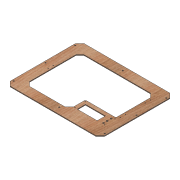
# Autodesk Inventor part: Front Face
Saved by Autodesk Inventor 2015 (Build 190159000, 159)
## iProperties
Created: 2018-04-12
Part Number: Front Face
Material: Wood (Birch)
Document SubType Name: Modeling
Designer: Ghassan Yusuf
Density: 0.55 g/cm^3
Appearance: Birch - Natural Polished
Author: Ghassan Yusuf
Autodesk Inventor part; units mm, degrees
ref_plane "YZ Plane" through (0, 0, 0) normal (1, 0, 0) x (0, 1, 0)
ref_plane "XZ Plane" through (0, 0, 0) normal (0, 1, 0) x (-1, 0, 0)
ref_plane "XY Plane" through (0, 0, 0) normal (0, 0, 1) x (1, 0, 0)
sketch "Faces Holing" plane through (0, 0, 0) normal (0, 0, 1) x (1, 0, 0)
  circle A0 centre (-222, 150) radius 3
  circle A1 centre (-222, 5) radius 3
  circle A2 centre (-222, -150) radius 3
  circle A3 centre (222, -150) radius 3
  circle A4 centre (222, 5) radius 3
  circle A5 centre (222, 150) radius 3
  circle A6 centre (0, 160) radius 3
  circle A7 centre (0, -150) radius 3
  point P0 (0, 2.5)
  dimension "d22" = 6
  dimension "d23" = 145
  dimension "d24" = 155
  measures "d22" diameter of A0
  measures "d23" distance of A4.centre A5.centre
  measures "d24" distance of A3.centre A4.centre
sketch "Hinges" plane through (0, 0, 0) normal (0, 0, 1) x (1, 0, 0)
  circle A0 centre (-439.8647, 121.4101) radius 1.75
  circle A1 centre (-439.8647, 95.9101) radius 1.75
  line L0 (-433.3647, 128.6601) -> (-449.3647, 128.6601)
  line L1 (-449.3647, 128.6601) -> (-449.3647, 88.6601)
  line L2 (-449.3647, 88.6601) -> (-433.3647, 88.6601)
  line L3 (-433.3647, 88.6601) -> (-433.3647, 128.6601)
  circle A2 centre (-464.8647, 95.9101) radius 1.75
  circle A3 centre (-464.8647, 121.4101) radius 1.75
  line L4 (-471.3647, 88.6601) -> (-455.3647, 88.6601)
  line L5 (-455.3647, 88.6601) -> (-455.3647, 128.6601)
  line L6 (-455.3647, 128.6601) -> (-471.3647, 128.6601)
  line L7 (-471.3647, 128.6601) -> (-471.3647, 88.6601)
  point P0 (-452.3647, 108.6601)
  dimension "d35" = 3.5
  dimension "d36" = 25.5
  dimension "d37" = 6.5
  dimension "d38" = 40
  dimension "d39" = 7.25
  dimension "d40" = 16
  dimension "d41" = 3.5
  dimension "d42" = 25.5
  dimension "d43" = 6.5
  dimension "d44" = 40
  dimension "d45" = 7.25
  dimension "d46" = 16
  dimension "d47" = 38
  measures "d35" diameter of A0
  measures "d36" distance of A1.centre A0.centre
  measures "d37" distance from line of L3 A0.centre
  measures "d38" distance of L2.end L0.start
  measures "d39" distance from line of L2 A1.centre
  measures "d40" distance of L0.start L0.end
  measures "d41" diameter of A2
  measures "d42" distance of A3.centre A2.centre
  measures "d43" distance from line of L7 A2.centre
  measures "d44" distance of L6.end L4.start
  measures "d45" distance from line of L6 A3.centre
  measures "d46" distance of L4.start L4.end
  measures "d47" distance between parallel lines of L3 L7
sketch "LCD2004" plane through (0, 0, 0) normal (0, 0, 1) x (1, 0, 0)
  line L0 (36.575, 21.45) -> (-61.225, 21.45)
  line L1 (-61.225, 21.45) -> (-61.225, -19.15)
  line L2 (-61.225, -19.15) -> (36.575, -19.15)
  line L3 (36.575, -19.15) -> (36.575, 21.45)
  circle A0 centre (-72.4, 31.74) radius 1.7
  circle A1 centre (-72.4, -18.56) radius 1.7
  circle A2 centre (72.4, -18.56) radius 1.7
  circle A3 centre (72.4, 31.74) radius 1.7
  line L4 (59.475, -39.15) -> (79.475, -19.15)
  circle A4 centre (61.875, 23.63) radius 4
  circle A5 centre (61.875, 4.43) radius 4
  circle A6 centre (61.875, -13.37) radius 4
  line L5 (-79.475, -39.15) -> (59.475, -39.15)
  line L6 (79.475, -19.15) -> (79.475, 39.15)
  line L7 (79.475, 39.15) -> (-79.475, 39.15)
  line L8 (-79.475, 39.15) -> (-79.475, -39.15)
  line L9 (-79.475, -39.15) -> (79.475, 39.15) construction
  line L10 (79.475, -39.15) -> (-79.475, 39.15) construction
  line L11 (-60.925, 21.15) -> (36.275, 21.15)
  line L12 (36.275, 21.15) -> (36.275, -18.85)
  line L13 (36.275, -18.85) -> (-60.925, -18.85)
  line L14 (-60.925, -18.85) -> (-60.925, 21.15)
  line L15 (-60.925, 21.15) -> (36.275, -18.85) construction
  line L16 (36.275, 21.15) -> (-60.925, -18.85) construction
  point P0 (4.405, 0.2073)
  point P1 (-12.325, 1.15)
  dimension "d55" = 158.95
  dimension "d56" = 78.3
  dimension "d57" = 18.55
  dimension "d58" = 20.3
  dimension "d59" = 20
  dimension "d60" = 8
  dimension "d61" = 8
  dimension "d62" = 8
  dimension "d63" = 40
  dimension "d64" = 97.2
  dimension "d65" = 15.52
  dimension "d66" = 17.6
  dimension "d67" = 19.2
  dimension "d68" = 17.8
  dimension "d69" = 3.4
  dimension "d70" = 50.3
  dimension "d71" = 7.41
  dimension "d72" = 7.075
  dimension "d73" = 144.8
  dimension "d74" = 0.3
  dimension "d75" = 20
  measures "d55" distance of L6.end L7.end
  measures "d56" distance between parallel lines of L5 L7
  measures "d57" distance between parallel lines of L8 L14
  measures "d58" distance between parallel lines of L5 L13
  measures "d59" distance from line of L4.start L6
  measures "d60" diameter of A4
  measures "d61" diameter of A5
  measures "d62" diameter of A6
  measures "d63" distance between parallel lines of L13 L11
  measures "d64" distance between parallel lines of L12 L14
  measures "d65" distance from line of L7 A4.centre
  measures "d66" distance from line of L6 A4.centre
  measures "d67" distance of A5.centre A4.centre
  measures "d68" distance of A6.centre A5.centre
  measures "d69" diameter of A0
  measures "d70" distance of A1.centre A0.centre
  measures "d71" distance from line of L7 A0.centre
  measures "d72" distance from line of L8 A0.centre
  measures "d73" distance of A3.centre A0.centre
  measures "d74" distance between parallel lines of L11 L0
  measures "d75" distance from line of L5 L4.end
sketch "Door Shape" plane through (0, 0, 0) normal (0, 0, 1) x (1, 0, 0)
  line L0 (13.05, -134) -> (33.05, -114)
  line L1 (33.05, -114) -> (33.05, -55.7)
  line L2 (33.05, -55.7) -> (182, -55.7)
  line L3 (182, -55.7) -> (182, 113)
  line L4 (182, 113) -> (162, 133)
  line L5 (162, 133) -> (-162, 133)
  line L6 (-162, 133) -> (-182, 113)
  line L7 (-182, 113) -> (-182, -114)
  line L8 (-182, -114) -> (-162, -134)
  line L9 (-162, -134) -> (13.05, -134)
  point P0 (-8.285, -11.54)
sketch "Sketch1" plane through (0, 0, 0) normal (0, 0, 1) x (1, 0, 0)
  line L0 (-230, 180) -> (230, 180)
  line L1 (230, 180) -> (230, -180)
  line L2 (230, -180) -> (-230, -180)
  line L3 (-230, -180) -> (-230, 180)
  line L4 (-182, 133) -> (182, 133)
  line L5 (182, 133) -> (182, -49)
  line L6 (-18, -134) -> (-182, -134)
  line L7 (-182, -134) -> (-182, 133)
  line L8 (-18, -134) -> (33.05, -134)
  line L9 (182, -55.7) -> (182, -49)
  line L10 (33.05, -55.7) -> (182, -55.7)
  line L11 (33.05, -134) -> (33.05, -55.7)
  point P0 (0, 0)
  point P1 (0, 180)
  point P2 (-230, 0)
  point P3 (0, 133)
  dimension "d0" = 360
  dimension "d1" = 460
  dimension "d5" = 364
  dimension "d6" = 267
  dimension "d53" = 148.95
  dimension "d54" = 78.3
  constraints: 24 end point, 4 horizontal, 4 perpendicular, 3 midpoint, 3 parallel, 2 vertical alignment, 1 horizontal alignment
  measures "d0" distance of L2.end L0.start
  measures "d1" distance of L0.start L0.end
  measures "d5" distance between parallel lines of L5 L7
  measures "d6" distance between parallel lines of L6 L4
  measures "d53" distance between parallel lines of L9 L11
  measures "d54" distance between parallel lines of L8 L10
extrude "Extrusion1" add sketch "Sketch1" against normal blind 4
chamfer "Chamfer1" distance 20 angle 45 4 edges at (230, 180, -2) (-230, 180, -2) (-230, -180, -2) (230, -180, -2)
chamfer "Chamfer2" distance 20 angle 45 4 edges at (-182, -134, -2) (-182, 133, -2) (182, 133, -2) (33.05, -134, -2)
sketch "Sketch3" plane through (0, 0, 0) normal (0, 0, 1) x (1, 0, 0)
  line L0 (210, -180) -> (-210, -180) projected
  line L1 (-230, -160) -> (-230, 160) projected
  line L2 (230, -160) -> (230, 160) projected
  line L3 (-210, 180) -> (210, 180) projected
  circle A0 centre (-222, 150) radius 3
  circle A1 centre (-222, 5) radius 3
  circle A2 centre (-222, -150) radius 3
  circle A3 centre (222, -150) radius 3
  circle A4 centre (222, 5) radius 3
  circle A5 centre (222, 150) radius 3
  circle A6 centre (0, 160) radius 3
  circle A7 centre (0, -150) radius 3
  point P0 (0, 0)
  dimension "d25" = 30
  dimension "d29" = 30
  dimension "d30" = 20
  dimension "d31" = 230
  dimension "d32" = 230
  measures "d31" distance of the line from the sketch origin of L1
  measures "d32" distance of the line from the sketch origin of L1
extrude "Extrusion3" cut sketch "Sketch3" against normal blind 46.25
sketch "Sketch4" plane through (0, 0, 0) normal (0, 0, 1) x (1, 0, 0)
  line L0 (-182, -114) -> (-182, 113) projected
  line L1 (182, -55.7) -> (182, 113) projected
  line L2 (33.05, -55.7) -> (182, -55.7) projected
  line L3 (162, 133) -> (-162, 133) projected
  circle A0 centre (191.5, 103.6789) radius 1.75
  circle A1 centre (191.5, 78.1789) radius 1.75
  line L4 (198, 110.9289) -> (182, 110.9289)
  line L5 (182, 110.9289) -> (182, 70.9289)
  line L6 (182, 70.9289) -> (198, 70.9289)
  line L7 (198, 70.9289) -> (198, 110.9289)
  circle A2 centre (166.5, 78.1789) radius 1.75
  circle A3 centre (166.5, 103.6789) radius 1.75
  line L8 (160, 70.9289) -> (176, 70.9289)
  line L9 (176, 70.9289) -> (176, 110.9289)
  line L10 (176, 110.9289) -> (160, 110.9289)
  line L11 (160, 110.9289) -> (160, 70.9289)
  circle A4 centre (191.5, -17.95) radius 1.75
  circle A5 centre (191.5, -43.45) radius 1.75
  line L12 (198, -10.7) -> (182, -10.7)
  line L13 (182, -10.7) -> (182, -50.7)
  line L14 (182, -50.7) -> (198, -50.7)
  line L15 (198, -50.7) -> (198, -10.7)
  circle A6 centre (166.5, -43.45) radius 1.75
  circle A7 centre (166.5, -17.95) radius 1.75
  line L16 (160, -50.7) -> (176, -50.7)
  line L17 (176, -50.7) -> (176, -10.7)
  line L18 (176, -10.7) -> (160, -10.7)
  line L19 (160, -10.7) -> (160, -50.7)
  circle A8 centre (-166.5, 12.75) radius 1.75
  circle A9 centre (-166.5, -12.75) radius 1.75
  line L20 (-160, 20) -> (-176, 20)
  line L21 (-176, 20) -> (-176, -20)
  line L22 (-176, -20) -> (-160, -20)
  line L23 (-160, -20) -> (-160, 20)
  circle A10 centre (-191.5, -12.75) radius 1.75
  circle A11 centre (-191.5, 12.75) radius 1.75
  line L24 (-198, -20) -> (-182, -20)
  line L25 (-182, -20) -> (-182, 20)
  line L26 (-182, 20) -> (-198, 20)
  line L27 (-198, 20) -> (-198, -20)
  point P0 (0, 0)
  point P1 (-182, -111.9289)
  point P2 (-182, 110.9289)
  point P3 (-160, 0)
  point P4 (182, 110.9289)
  point P5 (38.05, -55.7)
  point P6 (159.9289, 133)
  point P7 (-159.9289, 133)
  point P8 (182, -50.7)
  point P9 (177, -55.7)
  dimension "d77" = 5
  dimension "d81" = 10.7
  dimension "d82" = 70.9289
  dimension "d83" = 78.1789
  dimension "d84" = 17.95
  constraints: 3 vertical, 1 horizontal alignment, 2 other
extrude "Extrusion4" cut sketch "Sketch4" against normal blind 10 contours A0 | A1 | A4 | A5 | A10 | A11
fillet "Fillet2" radius 5 8 edges at (-210, -180, -2) (-230, -160, -2) (-230, 160, -2) (-210, 180, -2) (210, 180, -2) (230, 160, -2) (210, -180, -2) (230, -160, -2)
sketch "Sketch5" plane through (0, 0, 0) normal (0, 0, 1) x (1, 0, 0)
  line L0 (182, -55.7) -> (33.05, -55.7) projected
  line L1 (182, 113) -> (182, -55.7) projected
  line L2 (149.1, -73.4) -> (51.3, -73.4)
  line L3 (51.3, -73.4) -> (51.3, -114)
  line L4 (51.3, -114) -> (149.1, -114)
  line L5 (149.1, -114) -> (149.1, -73.4)
  circle A0 centre (40.125, -63.11) radius 1.7
  circle A1 centre (40.125, -113.41) radius 1.7
  circle A2 centre (184.925, -113.41) radius 1.7
  circle A3 centre (184.925, -63.11) radius 1.7
  line L6 (172, -134) -> (192, -114)
  circle A4 centre (174.4, -71.22) radius 4
  circle A5 centre (174.4, -90.42) radius 4
  circle A6 centre (174.4, -108.22) radius 4
  line L7 (33.05, -134) -> (172, -134)
  line L8 (192, -114) -> (192, -55.7)
  line L9 (192, -55.7) -> (33.05, -55.7)
  line L10 (33.05, -55.7) -> (33.05, -134)
  line L11 (33.05, -134) -> (192, -55.7) construction
  line L12 (192, -134) -> (33.05, -55.7) construction
  line L13 (51.6, -73.7) -> (148.8, -73.7)
  line L14 (148.8, -73.7) -> (148.8, -113.7)
  line L15 (148.8, -113.7) -> (51.6, -113.7)
  line L16 (51.6, -113.7) -> (51.6, -73.7)
  line L17 (51.6, -73.7) -> (148.8, -113.7) construction
  line L18 (148.8, -73.7) -> (51.6, -113.7) construction
  point P0 (0, 0)
  point P1 (38.05, -55.7)
  point P2 (182, 110.9289)
  point P3 (177, -55.7)
  point P4 (182, -50.7)
  dimension "d76" = 10
  constraints: 1 horizontal
extrude "Extrusion5" cut sketch "Sketch5" against normal blind 22.75 contours L5 L4 L3 L2 | A0 | A1 | A2 | A3 | A4 | A5 | A6 | L13 L14 L15 L16
fillet "Fillet3" radius 5 10 edges at (-182, -114, -2) (-182, 113, -2) (-162, -134, -2) (13.05, -134, -2) (33.05, -114, -2) (33.05, -55.7, -2) (182, -55.7, -2) (182, 113, -2) (-162, 133, -2) (162, 133, -2)
equation "\"d39\" = -0.5 * d36 + 0.5 * d38"
equation "\"d45\" = -0.5 * d42 + 0.5 * d44"
equation "\"d61\" = d60"
equation "\"d62\" = d60"
body "Solid1"
